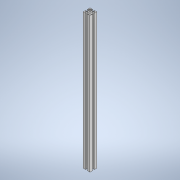
# Autodesk Inventor part: Part2
Saved by Autodesk Inventor 2022 (Build 260153000, 153)
## iProperties
Created: 2021-10-05
Part Number: Part2
Material: Generic
Document SubType Name: Modeling
Designer: Administrator
Density: 1 g/cm^3
Appearance: Default
Mass: 70.9377 g
Surface Area: 724.12 cm^2
Volume: 70.9377 cm^3
Author: Administrator
Autodesk Inventor part; units mm, degrees
ref_plane "YZ Plane" through (0, 0, 0) normal (1, 0, 0) x (0, 1, 0)
ref_plane "XZ Plane" through (0, 0, 0) normal (0, 1, 0) x (-1, 0, 0)
ref_plane "XY Plane" through (0, 0, 0) normal (0, 0, 1) x (1, 0, 0)
sketch "Sketch1" plane through (0, 0, 0) normal (0, 1, 0) x (-1, 0, 0)
  line L0 (-60.4078, 0.8339) -> (-63.4685, -2.2268)
  line L1 (-54.8385, -5.1661) -> (-54.8385, -3.6661)
  line L2 (-67.4685, 14.8339) -> (-67.4685, 7.4639)
  line L3 (-63.4685, 11.8946) -> (-60.4078, 8.8339)
  line L4 (-54.5291, 8.8339) -> (-51.4685, 11.8946)
  line L5 (-50.4078, 10.8339) -> (-53.4685, 7.7732)
  line L6 (-60.0985, 14.8339) -> (-67.4685, 14.8339)
  line L7 (-48.9685, 2.2039) -> (-47.4685, 2.2039)
  line L8 (-64.5291, -1.1661) -> (-61.4685, 1.8946)
  line L9 (-65.9685, 7.4639) -> (-67.4685, 7.4639)
  line L10 (-47.4685, 14.8339) -> (-54.8385, 14.8339)
  line L11 (-51.4685, -2.2268) -> (-54.5291, 0.8339)
  line L12 (-60.0985, 13.3339) -> (-63.4685, 13.3339)
  line L13 (-51.4685, 13.3339) -> (-54.8385, 13.3339)
  line L14 (-60.0985, -3.6661) -> (-60.0985, -5.1661)
  line L15 (-48.9685, 7.4639) -> (-48.9685, 10.8339)
  line L16 (-50.4078, -1.1661) -> (-48.9685, -1.1661)
  line L17 (-65.9685, 2.2039) -> (-65.9685, -1.1661)
  line L18 (-64.5291, 10.8339) -> (-65.9685, 10.8339)
  line L19 (-67.4685, -5.1661) -> (-60.0985, -5.1661)
  line L20 (-54.8385, -3.6661) -> (-51.4685, -3.6661)
  line L21 (-63.4685, -2.2268) -> (-63.4685, -3.6661)
  line L22 (-54.8385, -5.1661) -> (-47.4685, -5.1661)
  line L23 (-60.4078, 8.8339) -> (-54.5291, 8.8339)
  line L24 (-67.4685, 2.2039) -> (-67.4685, -5.1661)
  line L25 (-53.4685, 7.7732) -> (-53.4685, 1.8946)
  line L26 (-61.4685, 1.8946) -> (-61.4685, 7.7732)
  line L27 (-47.4685, -5.1661) -> (-47.4685, 2.2039)
  line L28 (-54.5291, 0.8339) -> (-60.4078, 0.8339)
  line L29 (-54.8385, 13.3339) -> (-54.8385, 14.8339)
  line L30 (-63.4685, 13.3339) -> (-63.4685, 11.8946)
  line L31 (-48.9685, 10.8339) -> (-50.4078, 10.8339)
  line L32 (-48.9685, -1.1661) -> (-48.9685, 2.2039)
  line L33 (-47.4685, 7.4639) -> (-47.4685, 14.8339)
  line L34 (-65.9685, -1.1661) -> (-64.5291, -1.1661)
  line L35 (-65.9685, 10.8339) -> (-65.9685, 7.4639)
  line L36 (-51.4685, -3.6661) -> (-51.4685, -2.2268)
  line L37 (-63.4685, -3.6661) -> (-60.0985, -3.6661)
  line L38 (-60.0985, 14.8339) -> (-60.0985, 13.3339)
  line L39 (-51.4685, 11.8946) -> (-51.4685, 13.3339)
  line L40 (-47.4685, 7.4639) -> (-48.9685, 7.4639)
  line L41 (-53.4685, 1.8946) -> (-50.4078, -1.1661)
  line L42 (-67.4685, 2.2039) -> (-65.9685, 2.2039)
  line L43 (-61.4685, 7.7732) -> (-64.5291, 10.8339)
  constraints: 88 end point, 32 equal length, 18 horizontal, 18 vertical, 8 collinear
extrude "Extrusion1" add sketch "Sketch1" along normal blind 400
sketch "Sketch2" plane through (0, 400, 0) normal (0, 1, 0) x (1, 0, 0)
  point P0 (57.4685, -4.8339)
hole "Hole1" at (57.4685, 400, 4.8339) direction (0, -1, 0) diameter 4 depth 400
body "Solid3"
